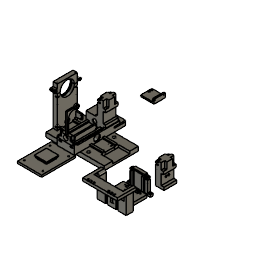
Lens_mount_movable_v1 (Autodesk Fusion 360 design; units mm, degrees)
part number: 2026-02-11-13-22-12-673
Autodesk Fusion 360 part; units mm, degrees
note: some values were not read from the file. Chosen so that the rebuilt part matches the saved one: which face or edge a step refers to. Set by a fixed rule: which sketch regions a step uses; the direction of a hole.
(part 1 of 4)
sketch "Sketch1" plane through (0, 0, 0) normal (0, 0, 1) x (1, 0, 0)
  line L0 (-175, 0) -> (-25, 0)
  line L1 (-25, -60) -> (-175, -60)
  line L2 (-175, 0) -> (-25, 0)
  line L3 (-175, -50) -> (-175, -55)
  line L4 (-190, -60) -> (-190, 0)
  line L5 (-175, 0) -> (-175, -60)
  line L6 (-25, -60) -> (-25, 0)
  line L7 (-25, -5) -> (-175, -5)
  line L8 (-175, -10) -> (-25, -10)
  line L9 (-25, -60) -> (15, -60)
  line L10 (15, -60) -> (15, 0)
  line L11 (15, 0) -> (-25, 0)
  line L12 (-25, 0) -> (-25, -60)
  line L13 (-175, -55) -> (-25, -55)
  line L14 (-190, 0) -> (-190, 5)
  line L15 (-190, 5) -> (-175, 5)
  line L16 (-175, 5) -> (-175, 0)
  line L17 (-175, -65) -> (-190, -65)
  line L18 (-190, -65) -> (-190, -60)
  line L19 (-175, -60) -> (-175, -65)
  line L20 (-190, -65) -> (-190, -70)
  line L21 (15, -70) -> (15, -60)
  line L22 (15, 0) -> (15, 10)
  line L23 (-190, 10) -> (-190, 5)
  line L24 (-175, -50) -> (-25, -50)
  line L25 (-190, -70) -> (-190, -90)
  line L26 (-190, -90) -> (15, -90)
  line L27 (15, -90) -> (15, -70)
  line L28 (15, 10) -> (15, 30)
  line L29 (15, 30) -> (-190, 30)
  line L30 (-190, 30) -> (-190, 10)
  point P0 (-175, 0)
  dimension "d236" = 60
  constraint horizontal L0
  constraint horizontal L1
  constraint horizontal L2
  constraint perpendicular L0 L6
  constraint coincident L6 L7.start
  constraint perpendicular L6 L7
  constraint coincident L5 L8.start
  constraint coincident L6 L8.end
  constraint perpendicular L6 L8
  constraint horizontal L9
  constraint vertical L10
  constraint horizontal L11
  constraint vertical L12
  constraint coincident L12 L13.end
  constraint perpendicular L12 L13
  constraint vertical L14
  constraint horizontal L15
  constraint vertical L16
  constraint coincident P0 L0.start
  constraint horizontal L17
  constraint vertical L18
  constraint vertical L19
  constraint perpendicular L17 L20
  constraint perpendicular L9 L21
  constraint perpendicular L11 L22
  constraint perpendicular L15 L23
  constraint coincident L6 L24.end
  constraint perpendicular L6 L24
  constraint parallel L20 L25
  constraint perpendicular L25 L26
  constraint perpendicular L26 L27
  constraint perpendicular L9 L28
  constraint perpendicular L28 L29
  constraint perpendicular L29 L30
  measures "d236" distance of L0 L1
sketch "Sketch11" plane through (0, 0, 0) normal (0, 0, 1) x (1, 0, 0)
  line L0 (-160, 89.8202) -> (-160, 19.8202)
  line L1 (-171.994, 80.8202) -> (-171.994, 28.8202)
  line L2 (-175, 89.8202) -> (-160, 89.8202)
  line L3 (-160, 70) -> (-160, 75)
  line L4 (-169.294, 28.8202) -> (-169.294, 80.8202)
  line L5 (-169.294, 80.8202) -> (-171.994, 80.8202)
  line L6 (-169.294, 28.8202) -> (-169.294, 80.8202)
  line L7 (-171.994, 28.8202) -> (-169.294, 28.8202)
  line L8 (-169.294, 80.8202) -> (-171.994, 80.8202)
  line L9 (-160, 19.8202) -> (-175, 19.8202)
  line L10 (-175, 89.8202) -> (-160, 89.8202)
  line L11 (-171.994, 80.8202) -> (-171.994, 28.8202)
  line L12 (-171.994, 28.8202) -> (-169.294, 28.8202)
  line L13 (-160, 19.8202) -> (-175, 19.8202)
  line L14 (-175, 19.8202) -> (-175, 89.8202)
  line L15 (-175, 30) -> (-175, 80)
  line L16 (-160, 35) -> (-160, 40)
  point P0 (-175, 80)
  point P1 (-175, 30)
  dimension "d76" = 2.7
  dimension "d77" = 9
  dimension "d78" = 9
  dimension "d79" = 2.7
  dimension "d80" = 9
  dimension "d81" = 9
  constraint vertical L15
  constraint vertical L16
  constraint vertical L3
  constraint horizontal L13
  constraint vertical L14
  constraint horizontal L2
  constraint vertical L0
  constraint horizontal L12
  constraint vertical L6
  constraint horizontal L5
  constraint vertical L1
  constraint horizontal L9
  constraint horizontal L10
  constraint horizontal L7
  constraint vertical L4
  constraint horizontal L8
  constraint vertical L11
  measures "d76" distance of L1.end L4.start
  measures "d77" distance of L2 L5
  measures "d78" distance of L12 L13
  measures "d79" distance of L1.end L4.start
  measures "d80" distance of L8 L10
  measures "d81" distance of L7 L9
extrude "Extrude19" add sketch "Sketch11" along normal blind 120 contours L1 L4 L5 L6 L7 L8 L11 L12 makes body 1
sketch "Sketch12" plane through (-169.294, 0, 0) normal (1, 0, 0) x (0, 1, 0)
  line L0 (80.849, 0) -> (80.849, 52.5)
  line L1 (28.849, 0) -> (80.849, 0)
  line L2 (80.0289, 0) -> (30.0289, 0)
  line L3 (80.849, 52.5) -> (28.849, 52.5)
  line L4 (28.849, 52.5) -> (28.849, 0)
  circle A0 centre (54.8202, 120) radius 26
  line L5 (28.8202, 0) -> (28.8202, 120)
  point P0 (80.0289, 0)
  dimension "d86" = 52
  dimension "d87" = 120
  measures "d86" diameter of A0
  measures "d87" distance of A0.centre L2
extrude "Extrude20" cut sketch "Sketch12" against normal blind 19.754 contours A0 bodies 1
extrude "Extrude21" add sketch "Sketch11" along normal blind 120 bodies 1
sketch "Sketch14" plane through (-160, 0, 0) normal (1, 0, 0) x (0, 1, 0)
  line L0 (19.8202, 0) -> (89.8202, 0)
  line L1 (89.8202, 0) -> (89.8202, 120)
  line L2 (89.8202, 120) -> (19.8202, 120)
  line L3 (19.8202, 120) -> (19.8202, 0)
  circle A0 centre (54.8202, 120) radius 25
  circle A1 centre (54.8202, 20.75) radius 5.5
  line L4 (89.8202, 0) -> (19.8202, 0)
  dimension "d98" = 50
  dimension "d99" = 11
  dimension "d100" = 20.75
  dimension "d1016" = 120
  measures "d98" diameter of A0
  measures "d99" diameter of A1
  measures "d100" distance of A1.centre L4
  measures "d1016" distance of A0.centre L4
extrude "Extrude25" cut sketch "Sketch14" against normal blind 58.28 contours L2 A0 picked at (62.4213, 115.1423) bodies 1
hole "Hole6" at (-160, 54.8202, 20.75) direction (-1, 0, 0) diameter 16 depth 25 tip angle 180 countersink diameter 17 countersink angle 30 bodies 1
sketch "Sketch29" plane through (0, 0, 0) normal (0, 0, 1) x (1, 0, 0)
  line L0 (45, 25) -> (100, 25)
  line L1 (100, 25) -> (100, 0)
  line L2 (100, 0) -> (45, 0)
  line L3 (45, 0) -> (45, 25)
  dimension "d216" = 55
  constraint horizontal L0
  constraint vertical L1
  constraint horizontal L2
  constraint vertical L3
  measures "d216" distance of L1.end L2.end
sketch "Sketch30" plane through (0, 0, 0) normal (0, -1, 0) x (1, 0, 0)
  line L0 (45, 0) -> (100, 0)
  line L1 (100, 0) -> (100, 20)
  line L2 (100, 20) -> (45, 20)
  line L3 (45, 20) -> (45, 0)
  line L4 (52.5, 5) -> (57.5, 5)
  line L5 (57.5, 5) -> (57.5, 0)
  line L6 (57.5, 0) -> (52.5, 0)
  line L7 (52.5, 0) -> (52.5, 5)
  line L8 (87.5, 5) -> (92.5, 5)
  line L9 (92.5, 5) -> (92.5, 0)
  line L10 (92.5, 0) -> (87.5, 0)
  line L11 (87.5, 0) -> (87.5, 5)
  circle A0 centre (72.5, 10) radius 7.5
  line L12 (52.5, 5) -> (51.5, 5)
  line L13 (51.5, 5) -> (52.5, 0)
  line L14 (57.5, 5) -> (58.5, 5)
  line L15 (58.5, 5) -> (57.5, 0)
  line L16 (87.5, 5) -> (86.5, 5)
  line L17 (86.5, 5) -> (87.5, 0)
  line L18 (92.5, 5) -> (93.5, 5)
  line L19 (93.5, 5) -> (92.5, 0)
  circle A1 centre (51.5, 5) radius 0.5
  circle A2 centre (58.5, 5) radius 0.5
  circle A3 centre (86.5, 5) radius 0.5
  circle A4 centre (93.5, 5) radius 0.5
  circle A5 centre (57.5, 0) radius 0.5
  circle A6 centre (52.5, 0) radius 0.5
  circle A7 centre (87.5, 0) radius 0.5
  circle A8 centre (92.5, 0) radius 0.5
  dimension "d215" = 30
  dimension "d217" = 7.5
  dimension "d218" = 15
  dimension "d219" = 10
  dimension "d220" = 1
  dimension "d221" = 1
  dimension "d222" = 1
  dimension "d223" = 1
  dimension "d224" = 1
  dimension "d225" = 1
  constraint horizontal L4
  constraint vertical L5
  constraint horizontal L6
  constraint vertical L7
  constraint coincident L0 L5.end
  constraint horizontal L8
  constraint vertical L9
  constraint horizontal L10
  constraint vertical L11
  constraint coincident L0 L9.end
  constraint perpendicular L7 L12
  constraint perpendicular L7 L14
  constraint perpendicular L11 L16
  constraint perpendicular L9 L18
  constraint coincident L12.end L13.start
  constraint coincident L14.end L15.start
  constraint coincident L16.end L17.start
  constraint coincident L18.end L19.start
  constraint coincident L5.end L6.start
  constraint coincident L6.end L7.start
  constraint coincident L10.end L11.start
  constraint coincident L9.end L10.start
  measures "d215" distance of L5 L11
  measures "d217" distance of L0.end L9.end
  measures "d218" diameter of A0
  measures "d219" distance of L0 A0.centre
  measures "d220" distance of L4.start L12.end
  measures "d221" distance of L4.end L14.end
  measures "d222" distance of L8.start L16.end
  measures "d223" distance of L8.end L18.end
  measures "d224" diameter of A1
  measures "d225" diameter of A2
extrude "Extrude46" add sketch "Sketch1" along normal blind 5 separate body contours L3 L4 L5 L14 L15 L16 L17 L18 L19 makes body 2
extrude "Extrude48" add sketch "Sketch1" along normal blind 10 contours L0 L2 L5 L6 L7 L12 | L5 L6 L8 L12 L24 | L3 L5 L6 L12 L13 L24 | L1 L5 L6 L12 L13 bodies 2
extrude "Extrude49" add sketch "Sketch1" along normal blind 15 contours L5 L6 L7 L8 L12 | L3 L5 L6 L12 L13 L24 bodies 2
extrude "Extrude50" add sketch "Sketch1" along normal blind 3 contours L6 L9 L10 L11 L12 bodies 2
extrude "Extrude51" add 2 faces at (-75, -6.6667, 15) (-75, -53.3333, 15) along direction (0, 0, 1) blind 5 on bodies 2 bodies 2
extrude "Extrude52" add 3 faces at (-75, -36.6667, 10) (-125, -58.3333, 10) (-125, -1.6667, 10) along direction (0, 0, 1) blind 5 on bodies 2 bodies 2
extrude "Extrude53" cut 1 faces at (-11.6667, -20, 3) along direction (0, 0, -1) blind 20.936 on bodies 2 bodies 2
extrude "Extrude54" add sketch "Sketch1" along normal blind 5 contours L6 L9 L10 L11 L12 bodies 2
sketch "Sketch31" plane through (-25, 0, 0) normal (1, 0, 0) x (0, 1, 0)
  line L0 (-60, 5) -> (0, 5)
  line L1 (0, 5) -> (0, 15)
  line L2 (0, 15) -> (-5, 15)
  line L3 (-5, 15) -> (-5, 20)
  line L4 (-5, 20) -> (-10, 20)
  line L5 (-10, 20) -> (-10, 15)
  line L6 (-50, 20) -> (-55, 20)
  line L7 (-55, 20) -> (-55, 15)
  line L8 (-55, 15) -> (-60, 15)
  line L9 (-60, 15) -> (-60, 5)
  circle A0 centre (-45.5, 12.25) radius 2
  circle A1 centre (-14.5, 12.25) radius 2
  line L10 (-45.5, 12.25) -> (-30, 12.25)
  line L11 (-30, 12.25) -> (-30, 27.75)
  circle A2 centre (-30, 27.75) radius 9.5
  line L12 (-10, 15) -> (-50, 15)
  line L13 (-50, 15) -> (-50, 20)
  dimension "d257" = 14.5
  dimension "d258" = 14.5
  dimension "d280" = 15.5
  dimension "d281" = 19
  constraint coincident A0.centre L10.start
  constraint horizontal L10
  constraint coincident L11.end A2.centre
  measures "d257" distance of L9 A0.centre
  measures "d258" distance of L1 A1.centre
  measures "d280" distance of L10.end L11.end
  measures "d281" diameter of A2
sketch "Sketch32" plane through (0, 0, 15) normal (0, 0, 1) x (-1, 0, 0)
  line L0 (25, 10) -> (175, 10)
  line L1 (175, 10) -> (175, 50)
  line L2 (25, 50) -> (25, 10)
  line L3 (35, 11.25) -> (33, 11.25)
  line L4 (33, 11.25) -> (33, 17.75)
  line L5 (33, 17.75) -> (35, 17.75)
  line L6 (35, 17.75) -> (35, 11.25)
  line L7 (25, 16.5) -> (25, 12.5)
  line L8 (25, 14.5) -> (41, 14.5)
  line L9 (35, 42.25) -> (33, 42.25)
  line L10 (33, 42.25) -> (33, 48.75)
  line L11 (33, 48.75) -> (35, 48.75)
  line L12 (35, 48.75) -> (35, 42.25)
  line L13 (25, 45.5) -> (41, 45.5)
  line L14 (175, 50) -> (25, 50)
  point P0 (25, 14.5)
  point P1 (25, 45.5)
  dimension "d271" = 6.5
  dimension "d273" = 10
  dimension "d274" = 2
  dimension "d275" = 2
  dimension "d276" = 6.5
  dimension "d277" = 10
  constraint horizontal L3
  constraint vertical L4
  constraint horizontal L5
  constraint vertical L6
  constraint coincident P0 L8.start
  constraint perpendicular L4 L8
  constraint midpoint L4 L8
  constraint horizontal L9
  constraint vertical L10
  constraint horizontal L11
  constraint vertical L12
  constraint coincident P1 L13.start
  constraint perpendicular L2 L13
  constraint midpoint L10 L13
  measures "d271" distance of L3.start L5.end
  measures "d273" distance of L6 L7
  measures "d274" distance of L4.end L5.end
  measures "d275" distance of L9.start L9.end
  measures "d276" distance of L9.start L11.end
  measures "d277" distance of L12 P1
hole "Hole8" at (-25, -45.5, 12.25) direction (-1, 0, 0) diameter 3 depth 20 tip angle 180 bodies 2
hole "Hole9" at (-25, -14.5, 12.25) direction (-1, 0, 0) diameter 3 depth 20 tip angle 180 bodies 2
extrude "Extrude55" cut 1 faces at (-11.6667, -20, 5) along direction (0, 0, -1) blind 9.616 on bodies 2 bodies 2
extrude "Extrude56" add sketch "Sketch1" along normal blind 6.6 contours L6 L9 L10 L11 L12 bodies 2
extrude "Extrude57" cut sketch "Sketch32" against normal blind 5.5 contours L3 L4 L6 L8 | L4 L5 L6 L8 | L9 L10 L12 L13 | L10 L11 L12 L13 bodies 2
sketch "Sketch34" plane through (-160, 0, 0) normal (1, 0, 0) x (0, 1, 0)
  line L0 (89.8202, 15) -> (81.0202, 15)
  line L1 (81.0202, 15) -> (81.0202, 17.5)
  line L2 (81.0202, 17.5) -> (89.8202, 17.5)
  line L3 (89.8202, 17.5) -> (89.8202, 15)
  line L4 (89.8202, 0) -> (19.8202, 0)
  line L5 (19.8202, 17.5) -> (28.6202, 17.5)
  line L6 (28.6202, 17.5) -> (28.6202, 15)
  line L7 (28.6202, 15) -> (19.8202, 15)
  line L8 (19.8202, 15) -> (19.8202, 17.5)
  line L9 (19.8202, 120) -> (19.8202, 0)
  line L10 (89.8202, 0) -> (89.8202, 120)
  dimension "d282" = 8.8
  dimension "d283" = 2.5
  dimension "d284" = 15
  dimension "d285" = 8.8
  dimension "d286" = 2.5
  dimension "d287" = 15
  dimension "d288" = 61.2
  dimension "d289" = 61.2
  constraint horizontal L0
  constraint vertical L1
  constraint horizontal L2
  constraint vertical L3
  constraint horizontal L5
  constraint vertical L6
  constraint horizontal L7
  constraint vertical L8
  measures "d282" distance of L0.start L0.end
  measures "d283" distance of L0.start L2.end
  measures "d284" distance of L0 L4
  measures "d285" distance of L5.start L5.end
  measures "d286" distance of L5.start L7.end
  measures "d287" distance of L4 L7
  measures "d288" distance of L1 L9
  measures "d289" distance of L6 L10
extrude "Extrude58" cut sketch "Sketch34" against normal blind 8 bodies 1
sketch "Sketch36" plane through (0, 0, 15) normal (0, 0, 1) x (-1, 0, 0)
  line L0 (160, -19.8202) -> (160, -28.6202)
  line L1 (160, -28.6202) -> (168, -28.6202)
  line L2 (168, -28.6202) -> (168, -19.8202)
  line L3 (168, -19.8202) -> (160, -19.8202)
  line L4 (164, -19.8202) -> (164, -24.2202)
  circle A0 centre (164, -24.2202) radius 2.5
  circle A1 centre (164, -24.2202) radius 4
  line L5 (164, -21.7202) -> (160, -21.7202)
  line L6 (164, -21.7202) -> (168, -21.7202)
  line L7 (164, -26.7202) -> (168, -26.7202)
  line L8 (164, -26.7202) -> (160, -26.7202)
  line L9 (160, -26.7202) -> (160, -21.7202)
  dimension "d292" = 4.4
  dimension "d293" = 5
  constraint midpoint L3 L4.start
  constraint perpendicular L1 L4
  constraint concentric A0 A1
  constraint coincident A0 L5.start
  constraint coincident L4 L5.start
  constraint coincident L0 L5.end
  constraint tangent A0 L5
  constraint perpendicular L0 L5
  constraint coincident L2 L6.end
  constraint tangent A0 L6
  constraint coincident A0 L7.start
  constraint coincident L2 L7.end
  constraint tangent A0 L7
  constraint perpendicular L2 L7
  constraint coincident L0 L8.end
  constraint tangent A0 L8
  measures "d292" distance of L4.start L4.end
  measures "d293" diameter of A0
extrude "Extrude59" cut sketch "Sketch36" against normal blind 16.922 contours A0 bodies 1
sketch "Sketch37" plane through (0, 0, 15) normal (0, 0, 1) x (-1, 0, 0)
  line L0 (160, -81.0202) -> (160, -89.8202)
  line L1 (160, -89.8202) -> (168, -89.8202)
  line L2 (168, -89.8202) -> (168, -81.0202)
  line L3 (168, -81.0202) -> (160, -81.0202)
  line L4 (160, -89.8202) -> (164, -89.8202)
  line L5 (164, -89.8202) -> (164, -85.4202)
  circle A0 centre (164, -85.4202) radius 4
  circle A1 centre (164, -85.4202) radius 2.5
  dimension "d296" = 5
  constraint coincident L0.end L1.start
  constraint midpoint L1 L4.end
  constraint perpendicular L4 L5
  constraint coincident L5.end A0.centre
  constraint tangent L0 A0
  measures "d296" diameter of A1
extrude "Extrude60" cut sketch "Sketch37" against normal blind 18.346 contours A1 bodies 1
extrude "Extrude75" cut sketch "Sketch36" along normal blind 10 contours A0 bodies 1
extrude "Extrude76" cut sketch "Sketch37" along normal blind 10 contours A1 bodies 1
extrude "Extrude61" add 1 faces at (-185, -36.6667, 5) along direction (0, 0, 1) blind 2 on bodies 2 bodies 2
extrude "Extrude63" add sketch "Sketch1" along normal blind 15 contours L0 L2 L11 L15 L16 L22 L23 L28 L29 L30 | L1 L9 L17 L19 L20 L21 L25 L26 L27 bodies 2
sketch "Sketch39" plane through (0, 0, 0) normal (0, 0, -1) x (1, 0, 0)
  line L0 (15, -30) -> (15, 90)
  line L1 (-190, 90) -> (-190, -30)
  line L2 (15, 90) -> (-190, 90)
  line L3 (-190, -30) -> (15, -30)
sketch "Sketch40" plane through (0, 0, 7) normal (0, 0, 1) x (-1, 0, 0)
  line L0 (175, 10) -> (175, 5)
  line L1 (175, -5) -> (190, -5)
  line L2 (190, -5) -> (190, 65)
  line L3 (190, 65) -> (175, 65)
  line L4 (175, 65) -> (175, 60)
  circle A0 centre (175, 65) radius 1
  circle A1 centre (175, -5) radius 1
  line L5 (175, 5) -> (175, -5)
  line L6 (175, 60) -> (175, 55)
  line L7 (175, 55) -> (175, 50)
  line L8 (175, 50) -> (175, 10)
  constraint coincident L3.end L4.start
  constraint coincident L1.start A1.centre
extrude "Extrude64" cut sketch "Sketch40" along normal blind 8.494 contours L3 L4 A0 picked at (175.2989, 65.5939) bodies 2
extrude "Extrude65" cut sketch "Sketch40" along normal blind 10.944 contours L1 A1 L5 | L1 A1 L5 bodies 2
sketch "Sketch41" plane through (0, 0, 0) normal (0, 0, 1) x (1, 0, 0)
  line L0 (-175, -65) -> (-179, -65)
  line L1 (-179, -65) -> (-179, -60.6)
  line L2 (-175, 5) -> (-179, 5)
  line L3 (-179, 5) -> (-179, 0.6)
  circle A0 centre (-179, -60.6) radius 2.5
  circle A1 centre (-179, 0.6) radius 2.5
  dimension "d311" = 4
  dimension "d312" = 4.4
  dimension "d313" = 4
  dimension "d314" = 4.4
  dimension "d315" = 5
  dimension "d316" = 5
  constraint horizontal L0
  constraint perpendicular L0 L1
  constraint horizontal L2
  constraint perpendicular L2 L3
  constraint coincident L1.end A0.centre
  constraint coincident L3.end A1.centre
  measures "d311" distance of L0.start L0.end
  measures "d312" distance of L0.end L1.end
  measures "d313" distance of L2.start L2.end
  measures "d314" distance of L2.end L3.end
  measures "d315" diameter of A0
  measures "d316" diameter of A1
hole "Hole10" at (-179, -60.6, 0) at (-179, 0.6, 0) direction (0, 0, 1) diameter 5 depth 10 tip angle 180 counterbore diameter 11 counterbore depth 4 bodies 2
sketch "Sketch42" plane through (-25, 0, 0) normal (1, 0, 0) x (0, 1, 0)
  line L0 (-60, 6.6) -> (0, 6.6)
  line L1 (0, 6.6) -> (0, 15)
  line L2 (0, 15) -> (-5, 15)
  line L3 (-5, 15) -> (-5, 20)
  line L4 (-5, 20) -> (-10, 20)
  line L5 (-10, 20) -> (-10, 15)
  line L6 (-50, 20) -> (-55, 20)
  line L7 (-55, 20) -> (-55, 15)
  line L8 (-55, 15) -> (-60, 15)
  line L9 (-60, 15) -> (-60, 6.6)
  circle A0 centre (-14.5, 12.25) radius 1.5
  circle A1 centre (-45.5, 12.25) radius 1.5
  line L10 (-10, 15) -> (-50, 15)
  line L11 (-50, 15) -> (-50, 20)
  line L12 (-50, 20) -> (-49, 20)
  line L13 (-49, 20) -> (-50, 15)
  line L14 (-55, 20) -> (-56, 20)
  line L15 (-56, 20) -> (-55, 15)
  line L16 (-10, 20) -> (-11, 20)
  line L17 (-11, 20) -> (-10, 15)
  line L18 (-5, 20) -> (-4, 20)
  line L19 (-4, 20) -> (-4.7712, 15)
  constraint coincident L6.start L11.end
  constraint perpendicular L11 L12
  constraint coincident L10.end L11.start
  constraint coincident L6.end L7.start
  constraint perpendicular L7 L14
  constraint coincident L7.end L8.start
  constraint coincident L4.end L5.start
  constraint perpendicular L5 L16
  constraint coincident L5.end L10.start
  constraint coincident L3.end L4.start
  constraint perpendicular L3 L18
  constraint coincident L2 L19.end
delete_face "DeleteFace2" [no effect]
extrude "Extrude66" cut sketch "Sketch40" along normal blind 10 contours L1 A1 L5 picked at (175.3187, -4.4164) bodies 2
extrude "Extrude67" add sketch "Sketch42" against normal blind 150 contours L7 L14 L15 | L2 L3 L18 L19 | L11 L12 L13 | L5 L16 L17 bodies 2
sketch "Sketch43" plane through (15, 0, 0) normal (1, 0, 0) x (0, 1, 0)
  line L0 (-90, 0) -> (30, 0)
  line L1 (30, 15) -> (0, 15)
  line L2 (0, 15) -> (0, 6.6)
  line L3 (0, 6.6) -> (-60, 6.6)
  line L4 (-60, 6.6) -> (-60, 15)
  line L5 (30, 0) -> (30, 15)
  line L6 (-60, 15) -> (-90, 15)
  line L7 (-90, 15) -> (-90, 0)
sketch "Sketch45" plane through (0, 0, 0) normal (0, 0, 1) x (1, 0, 0)
  line L0 (-25, 200) -> (-25, 80)
  line L1 (-35, 190) -> (-30, 190)
  line L2 (-30, 190) -> (-30, 80)
  line L3 (-30, 80) -> (-35, 80)
  line L4 (-35, 80) -> (-35, 190)
  line L5 (-25, 200) -> (-85, 200)
  line L6 (-85, 200) -> (-85, 80)
  line L7 (-85, 80) -> (-25, 80)
  line L8 (-80, 80) -> (-75, 80)
  line L9 (-75, 80) -> (-75, 190)
  line L10 (-75, 190) -> (-80, 190)
  line L11 (-80, 190) -> (-80, 80)
  constraint vertical L0
  constraint horizontal L1
  constraint vertical L2
  constraint horizontal L3
  constraint vertical L4
  constraint perpendicular L0 L5
  constraint perpendicular L5 L6
  constraint perpendicular L0 L7
  constraint horizontal L8
  constraint vertical L9
  constraint horizontal L10
  constraint vertical L11
  constraint coincident L7 L8.start
extrude "Extrude68" add sketch "Sketch45" along normal blind 25 separate body contours L0 L1 L2 L4 L5 L6 L7 L9 L10 L11 | L7 L8 L9 L10 L11 makes body 3
extrude "Extrude69" add sketch "Sketch45" along normal blind 30 contours L1 L2 L3 L4 L7 | L7 L8 L9 L10 L11 bodies 3
sketch "Sketch46" plane through (-25, 0, 0) normal (1, 0, 0) x (0, 1, 0)
  line L0 (80, 0) -> (200, 0)
  line L1 (200, 25) -> (80, 25)
  line L2 (80, 25) -> (80, 0)
  line L3 (115, 5) -> (120, 5)
  line L4 (120, 5) -> (120, 0)
  line L5 (120, 0) -> (115, 0)
  line L6 (115, 0) -> (115, 5)
  line L7 (160, 5) -> (165, 5)
  line L8 (165, 5) -> (165, 0)
  line L9 (165, 0) -> (160, 0)
  line L10 (160, 0) -> (160, 5)
  line L11 (120, 5) -> (121, 5)
  line L12 (121, 5) -> (120, 0)
  line L13 (115, 5) -> (114, 5)
  line L14 (114, 5) -> (115, 0)
  line L15 (160, 5) -> (159, 5)
  line L16 (159, 5) -> (160, 0)
  line L17 (165, 5) -> (166, 5)
  line L18 (166, 5) -> (165, 0)
  circle A0 centre (121, 5) radius 0.75
  circle A1 centre (114, 5) radius 0.75
  circle A2 centre (115, 0) radius 0.75
  circle A3 centre (120, 0) radius 0.75
  circle A4 centre (159, 5) radius 0.75
  circle A5 centre (166, 5) radius 0.75
  circle A6 centre (165, 0) radius 0.75
  circle A7 centre (160, 0) radius 0.75
  line L19 (120, 0) -> (140, 0)
  line L20 (140, 0) -> (140, 12.75)
  circle A8 centre (140, 12.75) radius 7.5
  line L21 (200, 0) -> (200, 25)
  line L22 (120.1471, 0.7354) -> (128.1471, 0.7354)
  line L23 (128.1471, 0.7354) -> (128.1507, 0)
  line L24 (159.8529, 0.7354) -> (151.8529, 0.7354)
  line L25 (151.8529, 0.7354) -> (151.8529, 0)
  dimension "d330" = 40
  dimension "d331" = 35
  dimension "d333" = 5
  dimension "d334" = 1.5
  dimension "d335" = 1.5
  dimension "d336" = 1.5
  dimension "d337" = 1.5
  dimension "d338" = 1.5
  dimension "d339" = 1.5
  dimension "d340" = 1.5
  dimension "d341" = 1.5
  dimension "d342" = 12.75
  dimension "d343" = 15
  dimension "d372" = 8
  dimension "d373" = 8
  dimension "d376" = 0.7354
  constraint horizontal L3
  constraint vertical L4
  constraint horizontal L5
  constraint vertical L6
  constraint coincident L0 L4.end
  constraint horizontal L7
  constraint vertical L8
  constraint horizontal L9
  constraint vertical L10
  constraint coincident L0 L8.end
  constraint perpendicular L4 L11
  constraint perpendicular L6 L13
  constraint perpendicular L10 L15
  constraint perpendicular L8 L17
  constraint coincident L11.end L12.start
  constraint coincident L13.end L14.start
  constraint coincident L5.end L6.start
  constraint coincident L4.end L5.start
  constraint coincident L15.end L16.start
  constraint coincident L17.end L18.start
  constraint coincident L8.end L9.start
  constraint coincident L9.end L10.start
  constraint midpoint L0 L19.end
  constraint perpendicular L19 L20
  constraint coincident L20.end A8.centre
  constraint coincident L12 L22.start
  constraint coincident A3 L22.start
  constraint horizontal L22
  constraint coincident L19 L23.end
  constraint coincident L16 L24.start
  constraint coincident A7 L24.start
  constraint perpendicular L10 L24
  constraint coincident L0 L25.end
  constraint perpendicular L0 L25
  measures "d330" distance of L4 L10
  measures "d331" distance of L2 L6
  measures "d333" distance of L8.end L9.end
  measures "d334" diameter of A0
  measures "d335" diameter of A1
  measures "d336" diameter of A2
  measures "d337" diameter of A3
  measures "d338" diameter of A4
  measures "d339" diameter of A5
  measures "d340" diameter of A6
  measures "d341" diameter of A7
  measures "d342" distance of L19.end L20.end
  measures "d343" diameter of A8
  measures "d372" distance of L22.start L22.end
  measures "d373" distance of L24.start L24.end
  measures "d376" vertical distance of L22.end L23.end
hole "Hole11" at (-25, 140, 12.75) direction (-1, 0, 0) diameter 13.9 depth 70.319 tip angle 180 countersink diameter 15 countersink angle 30 bodies 3
extrude "Extrude70" cut sketch "Sketch46" against normal blind 87.747 contours L0 L5 L6 A2 | L6 L14 A2 | L0 L14 A2 | L0 L3 L4 L5 L6 A2 A3 | L6 L13 L14 A1 A2 | L0 L4 L5 A3 | L13 L14 A1 | L13 L14 A1 | L0 L12 A3 L19 | L4 L12 A3 | L4 L11 L12 A0 A3 | L11 L12 A0 | L11 L12 A0 | L0 L18 A6 | L0 L16 A7 | L0 L8 L9 A6 | L8 L18 A6 | L8 L17 L18 A5 A6 | L0 L7 L8 L9 L10 A6 A7 | L0 L9 L10 A7 | L10 L16 A7 | L10 L15 L16 A4 A7 | L17 L18 A5 | L17 L18 A5 | L15 L16 A4 | L15 L16 A4 bodies 3
sketch "Sketch49" plane through (-85, 0, 0) normal (-1, 0, 0) x (0, -1, 0)
  arc A0 (-114.25, 0) -> (-114.8529, 0.7354) centre (-115, 0) ccw
  line L0 (-114.25, 0) -> (-80, 0)
  line L1 (-80, 0) -> (-80, 25)
  line L2 (-80, 25) -> (-200, 25)
  line L3 (-200, 25) -> (-200, 0)
  line L4 (-200, 0) -> (-165.75, 0)
  arc A1 (-165.1471, 0.7354) -> (-165.75, 0) centre (-165, 0) ccw
  line L5 (-165.1471, 0.7354) -> (-165.8529, 4.2646)
  arc A2 (-165.25, 5) -> (-165.8529, 4.2646) centre (-166, 5) ccw
  line L6 (-165.25, 5) -> (-159.75, 5)
  arc A3 (-159.1471, 4.2646) -> (-159.75, 5) centre (-159, 5) ccw
  line L7 (-159.1471, 4.2646) -> (-159.8529, 0.7354)
  arc A4 (-159.25, 0) -> (-159.8529, 0.7354) centre (-160, 0) ccw
  line L8 (-159.25, 0) -> (-120.75, 0)
  arc A5 (-120.1471, 0.7354) -> (-120.75, 0) centre (-120, 0) ccw
  line L9 (-120.1471, 0.7354) -> (-120.8529, 4.2646)
  arc A6 (-120.25, 5) -> (-120.8529, 4.2646) centre (-121, 5) ccw
  line L10 (-120.25, 5) -> (-114.75, 5)
  arc A7 (-114.1471, 4.2646) -> (-114.75, 5) centre (-114, 5) ccw
  line L11 (-114.1471, 4.2646) -> (-114.8529, 0.7354)
  circle A8 centre (-140, 12.75) radius 6.95
  line L12 (-140, 25) -> (-140, 12.75)
  circle A9 centre (-140, 12.75) radius 10
  dimension "d362" = 20
  constraint midpoint L2 L12.start
  constraint coincident A8.centre L12.end
  measures "d362" diameter of A9
hole "Hole12" at (-85, 140, 12.75) direction (1, 0, 0) diameter 21 depth 35 tip angle 180 bodies 3
sketch "Sketch51" plane through (0, 80, 0) normal (0, -1, 0) x (1, 0, 0)
  line L0 (-80, 25) -> (-85, 25)
  line L1 (-85, 25) -> (-85, 0)
  line L2 (-85, 0) -> (-25, 0)
  line L3 (-25, 0) -> (-25, 25)
  line L4 (-25, 25) -> (-30, 25)
  line L5 (-30, 25) -> (-30, 30)
  line L6 (-30, 30) -> (-35, 30)
  line L7 (-35, 30) -> (-35, 25)
  line L8 (-35, 25) -> (-75, 25)
  line L9 (-75, 25) -> (-75, 30)
  line L10 (-75, 30) -> (-80, 30)
  line L11 (-80, 30) -> (-80, 25)
  line L12 (-75, 30) -> (-74, 30)
  line L13 (-74, 30) -> (-75, 25)
  line L14 (-80, 30) -> (-81, 30)
  line L15 (-81, 30) -> (-80, 25)
  line L16 (-35, 30) -> (-36, 30)
  line L17 (-36, 30) -> (-35, 25)
  line L18 (-30, 30) -> (-29, 30)
  line L19 (-29, 30) -> (-30, 25)
  line L20 (-85, 22.25) -> (-70.5, 22.25)
  line L21 (-25, 22.25) -> (-39.5, 22.25)
  circle A0 centre (-70.5, 22.25) radius 1.5
  circle A1 centre (-39.5, 22.25) radius 1.5
  line L22 (-70.5, 22.25) -> (-55, 22.25)
  line L23 (-55, 22.25) -> (-55, 37.75)
  circle A2 centre (-55, 37.75) radius 9.5
  line L24 (-85, 16.6) -> (-25, 16.6)
  line L25 (-25, 11.6) -> (-85, 11.6)
  line L26 (-85, 16.6) -> (-85, 11.6)
  line L27 (-25, 16.6) -> (-25, 11.6)
  dimension "d366" = 14.5
  dimension "d367" = 14.5
  dimension "d368" = 3
  dimension "d369" = 3
  dimension "d370" = 2.75
  dimension "d371" = 2.75
  dimension "d377" = 15.5
  dimension "d378" = 19
  dimension "d398" = 5.65
  constraint coincident L9.end L10.start
  constraint perpendicular L9 L12
  constraint coincident L8.end L9.start
  constraint coincident L10.end L11.start
  constraint perpendicular L11 L14
  constraint coincident L0.start L11.end
  constraint coincident L6.end L7.start
  constraint perpendicular L7 L16
  constraint coincident L7.end L8.start
  constraint coincident L5.end L6.start
  constraint perpendicular L5 L18
  constraint coincident L4.end L5.start
  constraint coincident L1 L20.start
  constraint perpendicular L1 L20
  constraint coincident L3 L21.start
  constraint perpendicular L3 L21
  constraint coincident L20.end A0.centre
  constraint coincident L21.end A1.centre
  constraint parallel L20 L22
  constraint perpendicular L22 L23
  constraint coincident L23.end A2.centre
  constraint coincident L1 L24.start
  constraint coincident L3 L24.end
  constraint perpendicular L3 L24
  constraint coincident L3 L25.start
  constraint coincident L1 L25.end
  constraint perpendicular L1 L25
  measures "d366" distance of L20.start L20.end
  measures "d367" distance of L21.start L21.end
  measures "d368" diameter of A0
  measures "d369" diameter of A1
  measures "d370" distance of L8 L20.end
  measures "d371" distance of L8 L21.end
  measures "d377" distance of L22.end L23.end
  measures "d378" diameter of A2
  measures "d398" distance of L20.end L24
hole "Hole13" at (-70.5, 80, 22.25) at (-39.5, 80, 22.25) direction (0, 1, 0) diameter 3 depth 31 tip angle 180 bodies 3
sketch "Sketch52" plane through (0, 0, 25) normal (0, 0, 1) x (-1, 0, 0)
  line L0 (80, -80) -> (80, -190)
  line L1 (80, -190) -> (75, -190)
  line L2 (75, -190) -> (75, -80)
  line L3 (75, -80) -> (35, -80)
  line L4 (35, -80) -> (35, -190)
  line L5 (35, -190) -> (30, -190)
  line L6 (30, -190) -> (30, -80)
  line L7 (30, -80) -> (25, -80)
  line L8 (25, -80) -> (25, -200)
  line L9 (25, -200) -> (85, -200)
  line L10 (85, -200) -> (85, -80)
  line L11 (85, -80) -> (80, -80)
  line L12 (73.55, -91.6) -> (67.45, -91.6)
  line L13 (67.45, -91.6) -> (67.45, -90)
  line L14 (67.45, -90) -> (73.55, -90)
  line L15 (73.55, -90) -> (73.55, -91.6)
  line L16 (70.5, -80) -> (70.5, -85.95)
  line L17 (70.5, -85.95) -> (70.5, -97.25)
  line L18 (39.5, -80) -> (39.5, -103.2)
  line L19 (42.55, -91.6) -> (36.45, -91.6)
  line L20 (36.45, -91.6) -> (36.45, -90)
  line L21 (36.45, -90) -> (42.55, -90)
  line L22 (42.55, -90) -> (42.55, -91.6)
  point P0 (85, -80)
  point P1 (25, -80)
  dimension "d384" = 6.1
  dimension "d385" = 1.6
  dimension "d386" = 14.5
  dimension "d387" = 10
  dimension "d388" = 14.5
  dimension "d389" = 6.1
  dimension "d390" = 1.6
  dimension "d391" = 10
  constraint horizontal L12
  constraint vertical L13
  constraint horizontal L14
  constraint vertical L15
  constraint coincident L3 L16.start
  constraint perpendicular L3 L16
  constraint perpendicular L12 L17
  constraint midpoint L12 L17
  constraint coincident L3 L18.start
  constraint perpendicular L3 L18
  constraint horizontal L19
  constraint vertical L20
  constraint horizontal L21
  constraint vertical L22
  constraint midpoint L18 L19
  measures "d384" distance of L12.start L12.end
  measures "d385" distance of L12.start L14.end
  measures "d386" distance of L16.start P0
  measures "d387" distance of L3 L14
  measures "d388" distance of L18.start P1
  measures "d389" distance of L19.start L19.end
  measures "d390" distance of L19.start L21.end
  measures "d391" distance of L3 L21
extrude "Extrude72" cut sketch "Sketch46" against normal blind 74.394 contours L0 A3 L19 L22 L23 | L0 A7 L24 L25 bodies 3
extrude "Extrude73" add sketch "Sketch51" against normal blind 110 contours L11 L14 L15 | L9 L12 L13 | L7 L16 L17 | L5 L18 L19 bodies 3
extrude "Extrude74" cut sketch "Sketch52" against normal blind 5.6 contours L12 L14 L15 L17 | L12 L13 L14 L17 | L18 L19 L21 L22 | L18 L19 L20 L21 bodies 3
move_body "Move1" bodies 1 to x (1, 0, 0) y (0, 1, 0) z (0, 0, 1) at (0, 85, 0)
extrude "Extrude77" add sketch "Sketch51" along normal blind 20 contours L1 L3 L24 L25 L26 L27 bodies 3
sketch "Sketch55" plane through (0, 0, 0) normal (0, 0, 1) x (1, 0, 0)
  line L0 (25, 75) -> (85, 75)
  line L1 (85, 75) -> (85, 115)
  line L2 (85, 115) -> (25, 115)
  line L3 (25, 115) -> (25, 75)
  dimension "d432" = 60
  dimension "d433" = 40
  constraint horizontal L0
  constraint vertical L1
  constraint horizontal L2
  constraint vertical L3
  measures "d432" distance of L0.start L0.end
  measures "d433" distance of L0.start L2.end
extrude "Extrude79" add 1 faces at (-45, 200, 8.3333) along direction (0, 1, 0) blind 20 on bodies 3 bodies 3
extrude "Extrude80" add 2 faces at (-78.3333, 190, 28.3333) (-33.3333, 190, 28.3333) along direction (0, 1, 0) blind 20 on bodies 3 bodies 3
extrude "Extrude81" add 1 faces at (-65, 60, 14.9333) along direction (0, -1, 0) blind 20 on bodies 3 bodies 3
extrude "Extrude82" add sketch "Sketch51" along normal blind 20 contours L0 L1 L8 L9 L10 L11 L20 A0 L22 L23 | L11 L14 L15 | L1 L3 L4 L5 L6 L7 L8 L20 A0 L22 L23 L24 | L9 L12 L13 | L7 L16 L17 | L5 L18 L19 bodies 3
extrude "Extrude83" add sketch "Sketch51" along normal blind 40 contours L1 L2 L3 L25 bodies 3
sketch "Sketch56" plane through (0, 0, 25) normal (0, 0, 1) x (-1, 0, 0)
  line L0 (30, -210) -> (30, -60)
  line L1 (30, -60) -> (25, -60)
  line L2 (25, -60) -> (25, -220)
  line L3 (25, -220) -> (85, -220)
  line L4 (85, -220) -> (85, -60)
  line L5 (85, -60) -> (80, -60)
  line L6 (80, -60) -> (80, -210)
  line L7 (80, -210) -> (75, -210)
  line L8 (75, -210) -> (75, -60)
  line L9 (75, -60) -> (35, -60)
  line L10 (35, -60) -> (35, -210)
  line L11 (35, -210) -> (30, -210)
  line L12 (67.45, -91.6) -> (67.45, -90)
  line L13 (67.45, -90) -> (73.55, -90)
  line L14 (73.55, -90) -> (73.55, -91.6)
  line L15 (73.55, -91.6) -> (67.45, -91.6)
  line L16 (36.45, -91.6) -> (36.45, -90)
  line L17 (36.45, -90) -> (42.55, -90)
  line L18 (42.55, -90) -> (42.55, -91.6)
  line L19 (42.55, -91.6) -> (36.45, -91.6)
  line L20 (25, -220) -> (85, -220)
  line L21 (85, -220) -> (85, -210)
  line L22 (85, -210) -> (25, -210)
  line L23 (25, -210) -> (25, -220)
  constraint horizontal L20
  constraint vertical L21
  constraint horizontal L22
  constraint vertical L23
  constraint coincident L4 L21.end
  constraint coincident L2.end L3.start
sketch "Sketch57" plane through (0, 0, 25) normal (0, 0, 1) x (-1, 0, 0)
  line L0 (75, -210) -> (75, -60)
  line L1 (30, -60) -> (25, -60)
  line L2 (35, -60) -> (35, -210)
  line L3 (67.45, -91.6) -> (67.45, -90)
  line L4 (67.45, -90) -> (73.55, -90)
  line L5 (73.55, -90) -> (73.55, -91.6)
  line L6 (73.55, -91.6) -> (67.45, -91.6)
  line L7 (36.45, -91.6) -> (36.45, -90)
  line L8 (36.45, -90) -> (42.55, -90)
  line L9 (42.55, -90) -> (42.55, -91.6)
  line L10 (42.55, -91.6) -> (36.45, -91.6)
  line L11 (42.75, -72) -> (36.25, -72)
  line L12 (36.25, -72) -> (36.25, -70)
  line L13 (36.25, -70) -> (42.75, -70)
  line L14 (42.75, -70) -> (42.75, -72)
  line L15 (67.25, -70) -> (73.75, -70)
  line L16 (73.75, -70) -> (73.75, -72)
  line L17 (73.75, -72) -> (67.25, -72)
  line L18 (67.25, -72) -> (67.25, -70)
  line L19 (70.5, -60) -> (70.5, -80)
  line L20 (39.5, -60) -> (39.5, -80)
  line L21 (30, -210) -> (30, -60)
  line L22 (25, -60) -> (25, -220)
  line L23 (25, -220) -> (85, -220)
  line L24 (85, -220) -> (85, -60)
  line L25 (85, -60) -> (80, -60)
  line L26 (80, -60) -> (80, -210)
  line L27 (80, -210) -> (75, -210)
  line L28 (35, -210) -> (30, -210)
  line L29 (75, -60) -> (35, -60)
  dimension "d421" = 6.5
  dimension "d422" = 2
  dimension "d423" = 6.5
  dimension "d424" = 2
  dimension "d427" = 10
  dimension "d429" = 10
  dimension "d530" = 14.5
  dimension "d531" = 14.5
  constraint horizontal L11
  constraint vertical L12
  constraint horizontal L13
  constraint vertical L14
  constraint horizontal L17
  constraint vertical L18
  constraint horizontal L15
  constraint vertical L16
  constraint coincident L1 L19.start
  constraint perpendicular L1 L19
  constraint midpoint L15 L19
  constraint coincident L1 L20.start
  constraint midpoint L13 L20
  measures "d421" distance of L11.start L11.end
  measures "d422" distance of L11.start L13.end
  measures "d423" distance of L17.end L16.end
  measures "d424" distance of L15.end L16.end
  measures "d427" distance of L1 L15
  measures "d429" distance of L1 L13
  measures "d530" distance of L20 L22
  measures "d531" distance of L19 L24
extrude "Extrude85" cut sketch "Sketch57" against normal blind 5.6 contours L11 L13 L14 L20 | L11 L12 L13 L20 | L15 L17 L18 L19 | L15 L16 L17 L19 bodies 3
sketch "Sketch59" plane through (0, 75, 0) normal (0, -1, 0) x (1, 0, 0)
  line L0 (25, 0) -> (85, 0)
  line L1 (85, 0) -> (85, 25)
  line L2 (85, 25) -> (25, 25)
  line L3 (25, 25) -> (25, 0)
  line L4 (30, 0) -> (35, 0)
  line L5 (35, 0) -> (35, 5)
  line L6 (35, 5) -> (30, 5)
  line L7 (30, 5) -> (30, 0)
  line L8 (75, 0) -> (80, 0)
  line L9 (80, 0) -> (80, 5)
  line L10 (80, 5) -> (75, 5)
  line L11 (75, 5) -> (75, 0)
  line L12 (35, 5) -> (36, 5)
  line L13 (36, 5) -> (35, 0)
  line L14 (30, 5) -> (29, 5)
  line L15 (29, 5) -> (30, 0)
  line L16 (75, 5) -> (74, 5)
  line L17 (74, 5) -> (75, 0)
  line L18 (80, 5) -> (81, 5)
  line L19 (81, 5) -> (80, 0)
  circle A0 centre (36, 5) radius 1
  circle A1 centre (29, 5) radius 1
  circle A2 centre (35, 0) radius 1
  circle A3 centre (30, 0) radius 1
  circle A4 centre (74, 5) radius 1
  circle A5 centre (81, 5) radius 1
  circle A6 centre (80, 0) radius 1
  circle A7 centre (75, 0) radius 1
  circle A8 centre (55, 12.75) radius 7
  dimension "d442" = 5
  dimension "d443" = 5
  dimension "d444" = 5
  dimension "d445" = 5
  dimension "d446" = 5
  dimension "d447" = 5
  dimension "d448" = 2
  dimension "d449" = 2
  dimension "d450" = 2
  dimension "d451" = 2
  dimension "d452" = 2
  dimension "d453" = 2
  dimension "d454" = 2
  dimension "d455" = 2
  dimension "d456" = 30
  dimension "d457" = 12.75
  dimension "d470" = 14
  constraint horizontal L4
  constraint vertical L5
  constraint horizontal L6
  constraint vertical L7
  constraint coincident L0 L4.start
  constraint horizontal L8
  constraint vertical L9
  constraint horizontal L10
  constraint vertical L11
  constraint coincident L0 L8.start
  constraint perpendicular L5 L12
  constraint perpendicular L7 L14
  constraint perpendicular L11 L16
  constraint parallel L15 L17
  constraint perpendicular L9 L18
  constraint coincident L12.end L13.start
  constraint coincident L14.end L15.start
  constraint coincident L4.end L5.start
  constraint coincident L4.start L7.end
  constraint coincident L16.end L17.start
  constraint coincident L18.end L19.start
  constraint coincident L8.end L9.start
  constraint coincident L8.start L11.end
  measures "d442" distance of L4.start L4.end
  measures "d443" distance of L4.start L6.end
  measures "d444" distance of L8.start L8.end
  measures "d445" distance of L8.start L10.end
  measures "d446" distance of L3 L7
  measures "d447" distance of L1 L9
  measures "d448" diameter of A0
  measures "d449" diameter of A1
  measures "d450" diameter of A2
  measures "d451" diameter of A3
  measures "d452" diameter of A4
  measures "d453" diameter of A5
  measures "d454" diameter of A6
  measures "d455" diameter of A7
  measures "d456" distance of L3 A8.centre
  measures "d457" distance of L0 A8.centre
  measures "d470" diameter of A8
sketch "Sketch60" plane through (0, 115, 0) normal (0, 1, 0) x (-1, 0, 0)
  line L0 (-85, 0) -> (-25, 0)
  line L1 (-25, 0) -> (-25, 25)
  line L2 (-25, 25) -> (-85, 25)
  line L3 (-85, 25) -> (-85, 0)
  line L4 (-55, 0) -> (-55, 12.75)
  circle A0 centre (-55, 12.75) radius 10
  dimension "d458" = 12.75
  dimension "d459" = 20
  constraint midpoint L0 L4.start
  constraint perpendicular L0 L4
  constraint coincident L4.end A0.centre
  measures "d458" distance of L4.start L4.end
  measures "d459" diameter of A0
hole "Hole18" at (-85, 140, 12.75) direction (1, 0, 0) diameter 23 depth 3 tip angle 180 bodies 3
sketch "Sketch61" plane through (0, 0, 0) normal (0, 0, 1) x (1, 0, 0)
  line L0 (-80.0135, 225) -> (-30.0135, 225)
  line L1 (-30.0135, 225) -> (-30.0135, 235)
  line L2 (-30.0135, 235) -> (-80.0135, 235)
  line L3 (-80.0135, 235) -> (-80.0135, 225)
  circle A0 centre (-32.5135, 232.5) radius 2.5
  circle A1 centre (-77.5135, 232.5) radius 2.5
  dimension "d486" = 50
  dimension "d489" = 5
  dimension "d490" = 7.5
  dimension "d491" = 2.5
  dimension "d492" = 5
  dimension "d493" = 7.5
  dimension "d494" = 2.5
  constraint horizontal L0
  constraint vertical L1
  constraint horizontal L2
  constraint vertical L3
  measures "d486" distance of L1 L3
  measures "d489" diameter of A0
  measures "d490" distance of L0 A0.centre
  measures "d491" distance of L1 A0.centre
  measures "d492" diameter of A1
  measures "d493" distance of L0 A1.centre
  measures "d494" distance of L3 A1.centre
extrude "Extrude88" add sketch "Sketch61" along normal blind 23 separate body makes body 4
sketch "Sketch62" plane through (0, 235, 0) normal (0, 1, 0) x (-1, 0, 0)
  line L0 (30.0135, 0) -> (80.0135, 0)
  line L1 (80.0135, 0) -> (80.0135, 23)
  line L2 (80.0135, 23) -> (30.0135, 23)
  line L3 (30.0135, 23) -> (30.0135, 0)
  line L4 (55.0135, 0) -> (55.0135, 12.75)
  circle A0 centre (55.0135, 12.75) radius 8
  dimension "d479" = 12.75
  dimension "d480" = 16
  constraint midpoint L0 L4.start
  constraint perpendicular L0 L4
  constraint coincident L4.end A0.centre
  measures "d479" distance of L4.start L4.end
  measures "d480" diameter of A0
hole "Hole20" at (-55.0135, 235, 12.75) direction (0, -1, 0) diameter 16 depth 10 tip angle 180 countersink diameter 17 countersink angle 30 bodies 4
sketch "Sketch63" plane through (0, 0, 25) normal (0, 0, 1) x (-1, 0, 0)
  line L0 (42.75, -72) -> (36.25, -72)
  line L1 (25, -60) -> (25, -220)
  line L2 (25, -220) -> (85, -220)
  line L3 (85, -220) -> (85, -60)
  line L4 (30, -60) -> (25, -60)
  line L5 (80, -60) -> (80, -210)
  line L6 (80, -210) -> (75, -210)
  line L7 (75, -210) -> (75, -60)
  line L8 (75, -60) -> (35, -60)
  line L9 (35, -60) -> (35, -210)
  line L10 (35, -210) -> (30, -210)
  line L11 (30, -210) -> (30, -60)
  line L12 (67.45, -91.6) -> (67.45, -90)
  line L13 (67.45, -90) -> (73.55, -90)
  line L14 (73.55, -90) -> (73.55, -91.6)
  line L15 (73.55, -91.6) -> (67.45, -91.6)
  line L16 (36.45, -91.6) -> (36.45, -90)
  line L17 (36.45, -90) -> (42.55, -90)
  line L18 (42.55, -90) -> (42.55, -91.6)
  line L19 (42.55, -91.6) -> (36.45, -91.6)
  line L20 (25, -220) -> (30, -220)
  line L21 (30, -220) -> (30, -210)
  line L22 (30, -210) -> (25, -210)
  line L23 (25, -210) -> (25, -220)
  line L24 (80, -210) -> (85, -210)
  line L25 (85, -210) -> (85, -220)
  line L26 (85, -220) -> (80, -220)
  line L27 (80, -220) -> (80, -210)
  circle A0 centre (75, -216) radius 2.5
  circle A1 centre (35, -216) radius 2.5
  line L28 (36.25, -72) -> (36.25, -70)
  line L29 (36.25, -70) -> (42.75, -70)
  line L30 (42.75, -70) -> (42.75, -72)
  line L31 (73.75, -70) -> (73.75, -72)
  line L32 (73.75, -72) -> (67.25, -72)
  line L33 (67.25, -72) -> (67.25, -70)
  line L34 (67.25, -70) -> (73.75, -70)
  line L35 (85, -60) -> (80, -60)
  dimension "d507" = 5
  dimension "d508" = 5
  dimension "d518" = 4
  dimension "d519" = 4
  constraint horizontal L20
  constraint vertical L21
  constraint horizontal L22
  constraint vertical L23
  constraint coincident L10.end L11.start
  constraint coincident L1.end L2.start
  constraint horizontal L24
  constraint vertical L25
  constraint horizontal L26
  constraint vertical L27
  constraint coincident L2.end L3.start
  constraint coincident L5.end L6.start
  measures "d507" diameter of A0
  measures "d508" diameter of A1
  measures "d518" distance of L2 A1.centre
  measures "d519" distance of L2 A0.centre
extrude "Extrude89" add sketch "Sketch63" along normal blind 5 contours L1 L2 L20 L21 L22 L23 | L2 L3 L24 L25 L26 L27 bodies 3
extrude "Extrude90" cut sketch "Sketch61" along normal blind 25.255 contours L1 L2 A0 bodies 4
extrude "Extrude91" cut sketch "Sketch61" along normal blind 24.513 contours L2 L3 A1 bodies 4
sketch "Sketch64" plane through (0, 0, 23) normal (0, 0, 1) x (-1, 0, 0)
  arc A0 (77.5135, -235) -> (80.0135, -232.5) centre (77.5135, -232.5) ccw
  line L0 (80.0135, -232.5) -> (80.0135, -225)
  line L1 (80.0135, -225) -> (30.0135, -225)
  line L2 (30.0135, -225) -> (30.0135, -232.5)
  arc A1 (30.0135, -232.5) -> (32.5135, -235) centre (32.5135, -232.5) ccw
  line L3 (32.5135, -235) -> (77.5135, -235)
  circle A2 centre (35.0135, -230) radius 4.5
  circle A3 centre (75, -230) radius 4.5
  line L4 (70.5, -230) -> (70.5, -225)
  line L5 (79.1119, -231.8282) -> (80.0135, -231.8282)
  line L6 (30.9016, -231.8282) -> (30.0135, -231.8282)
  line L7 (39.5133, -229.9603) -> (39.4696, -225)
  dimension "d499" = 9
  dimension "d500" = 9
  constraint coincident A3 L4.start
  constraint coincident L1 L4.end
  constraint perpendicular L1 L4
  constraint coincident A3 L5.start
  constraint coincident L0 L5.end
  constraint perpendicular L0 L5
  constraint coincident A2 L6.start
  constraint coincident L2 L6.end
  constraint perpendicular L2 L6
  constraint coincident A2 L7.start
  constraint coincident L1 L7.end
  constraint tangent A2 L7
  measures "d499" diameter of A2
  measures "d500" diameter of A3
extrude "Extrude179" cut sketch "Sketch64" against normal blind 13 contours L0 L1 A3 L4 L5 | A3 | L1 L2 A2 L6 L7 | A2 bodies 4
sketch "Sketch65" plane through (0, 0, 10) normal (0, 0, 1) x (-1, 0, 0)
  line L0 (80.0135, -232.5) -> (80.0135, -225)
  line L1 (80.0135, -225) -> (62.526, -225)
  line L2 (63.0563, -235) -> (77.5135, -235)
  arc A0 (77.5135, -235) -> (80.0135, -232.5) centre (77.5135, -232.5) ccw
  circle A1 centre (75, -229) radius 2.5
  line L3 (80.0135, -225) -> (30.0135, -225)
  line L4 (62.526, -225) -> (62.526, -233.134)
  spline S0 degree 2 poles (63.0563, -235) (62.7831, -234.0352) (62.526, -233.134) knots 0 0 0 0.193993 0.193993 0.193993 weights 1 1.000517 1
  dimension "d503" = 5
  dimension "d517" = 4
  measures "d503" diameter of A1
  measures "d517" distance of A1.centre L3
sketch "Sketch66" plane through (0, 0, 10) normal (0, 0, 1) x (-1, 0, 0)
  line L0 (47.501, -225) -> (30.0135, -225)
  line L1 (30.0135, -225) -> (30.0135, -232.5)
  arc A0 (30.0135, -232.5) -> (32.5135, -235) centre (32.5135, -232.5) ccw
  line L2 (32.5135, -235) -> (46.9706, -235)
  circle A1 centre (35, -229) radius 2.5
  line L3 (80.0135, -225) -> (30.0135, -225)
  line L4 (47.501, -233.134) -> (47.501, -225)
  spline S0 degree 2 poles (47.501, -233.134) (47.2438, -234.0352) (46.9706, -235) knots 0 0 0 0.193993 0.193993 0.193993 weights 1 1.000517 1
  dimension "d504" = 5
  dimension "d516" = 4
  measures "d504" diameter of A1
  measures "d516" distance of A1.centre L3
hole "Hole21" at (-75, 229, 10) at (-35, 229, 10) direction (0, 0, -1) diameter 5 depth 34.895 tip angle 180 bodies 4
hole "Hole22" at (-35, 216, 25) at (-75, 216, 25) direction (0, 0, -1) diameter 5 depth 25 tip angle 180 bodies 3